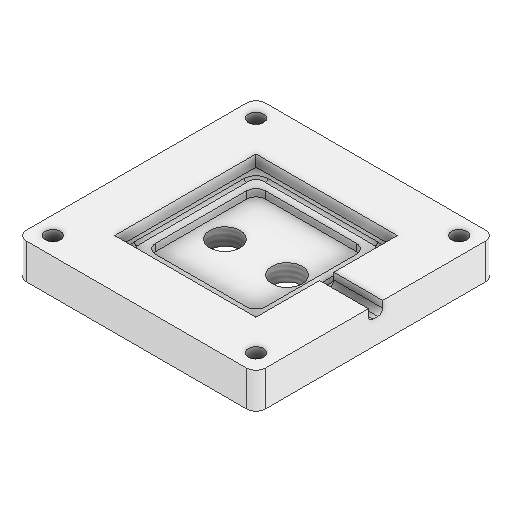
# Autodesk Inventor part: inf_soporte
Saved by Autodesk Inventor 2026.2 (Build 302298010, 298A)
## iProperties
Created: 2026-04-29
Part Number: inf_soporte
Material: Generic
Document SubType Name: Modeling
Designer: danie
Density: 1 g/cm^3
Appearance: Default
Author: danie
Autodesk Inventor part; units mm, degrees
ref_plane "YZ Plane" through (0, 0, 0) normal (1, 0, 0) x (0, 1, 0)
ref_plane "XZ Plane" through (0, 0, 0) normal (0, 1, 0) x (-1, 0, 0)
sketch "peltier" plane through (0, 0, 0) normal (0, 0, 1) x (1, 0, 0)
  line L0 (7.1779, -44.0485) -> (-50.9721, -44.0485)
  line L1 (-50.9721, -44.0485) -> (-50.9721, -102.2985)
  line L2 (-50.9721, -102.2985) -> (7.1779, -102.2985)
  line L3 (7.1779, -102.2985) -> (7.1779, -44.0485)
  point P0 (-21.8971, -73.1735)
  point P1 (-21.8971, -73.1735)
  dimension "d0" = 58.25
  dimension "d1" = 58.15
  measures "d0" distance between parallel lines of L2 L0
  measures "d1" distance between parallel lines of L3 L1
sketch "Sketch1" plane through (0, 0, 0) normal (0, 1, 0) x (-1, 0, 0)
  line L0 (-46, 50) -> (46, 50)
  line L1 (50, 46) -> (50, -46)
  line L2 (46, -50) -> (-46, -50)
  line L3 (-50, -46) -> (-50, 46)
  line L4 (-50, 50) -> (50, -50) construction
  line L5 (50, 50) -> (-50, -50) construction
  line L6 (-29.575, 29.575) -> (29.575, 29.575)
  line L7 (29.575, 29.575) -> (29.575, -29.575)
  line L8 (29.575, -29.575) -> (-29.575, -29.575)
  line L9 (-29.575, -29.575) -> (-29.575, 29.575)
  line L10 (-29.575, 29.575) -> (29.575, -29.575) construction
  line L11 (29.575, 29.575) -> (-29.575, -29.575) construction
  line L12 (-29.575, 0) -> (-50, 0)
  line L13 (-19, 23) -> (19, 23)
  line L14 (23, 19) -> (23, -19)
  line L15 (19, -23) -> (-19, -23)
  line L16 (-23, -19) -> (-23, 19)
  line L17 (-23, 23) -> (23, -23) construction
  line L18 (23, 23) -> (-23, -23) construction
  arc A0 (50, 46) -> (46, 50) centre (46, 46) ccw
  arc A1 (-46, 50) -> (-50, 46) centre (-46, 46) ccw
  arc A2 (-50, -46) -> (-46, -50) centre (-46, -46) ccw
  arc A3 (46, -50) -> (50, -46) centre (46, -46) ccw
  arc A4 (23, 19) -> (19, 23) centre (19, 19) ccw
  arc A5 (-19, 23) -> (-23, 19) centre (-19, 19) ccw
  arc A6 (-23, -19) -> (-19, -23) centre (-19, -19) ccw
  arc A7 (19, -23) -> (23, -19) centre (19, -19) ccw
  line L19 (-29.575, 0) -> (-29.575, -3)
  line L20 (-29.575, -3) -> (-50, -3)
  line L21 (-50, -3) -> (-50, 3)
  line L22 (-50, 3) -> (-29.575, 3)
  line L23 (-29.575, 3) -> (-29.575, -3)
  circle A8 centre (13, 0) radius 6.35
  circle A9 centre (-13, 0) radius 6.35
  line L24 (29.075, 29.125) -> (-29.075, 29.125)
  line L25 (-29.075, 29.125) -> (-29.075, -29.125)
  line L26 (-29.075, -29.125) -> (29.075, -29.125)
  line L27 (29.075, -29.125) -> (29.075, 29.125)
  point P0 (0, 0)
  point P1 (0, 0)
  dimension "d2" = 100
  dimension "d3" = 100
  dimension "d4" = 0.5
  dimension "d5" = 4
  dimension "d6" = 46
  dimension "d7" = 46
  dimension "d8" = 4
  dimension "d13" = 3
  dimension "d14" = 6
  dimension "d17" = 12.7
  dimension "d18" = 13
  dimension "d19" = 13
  dimension "d20" = 12.7
  constraints: 48 end point, 21 point on line, 16 point on circle, 16 tangent, 10 centre point, 8 midpoint, 6 equal radius, 6 parallel, 6 perpendicular, 3 horizontal, 2 other
  measures "d2" distance between parallel lines of L3 L1
  measures "d3" distance between parallel lines of L2 L0
  measures "d5" radius of A0
  measures "d6" distance between parallel lines of L16 L14
  measures "d7" distance between parallel lines of L13 L15
  measures "d8" radius of A4
  measures "d13" distance of L12.start L19.end
  measures "d14" distance of L20.end L21.end
  measures "d17" diameter of A8
  measures "d20" diameter of A9
extrude "Extrusion1" add sketch "Sketch1" along normal blind 20 contours L0 A0 L1 A3 L2 A2 L3 L20 L9 L8 L7 L6 L22 A1
extrude "Extrusion2" add sketch "Sketch1" along normal blind 15 contours L22 L9 L12 L3 | L12 L9 L20 L3 | L9 L6 L7 L8 | L27 L26 L25 L24
extrude "Extrusion3" add sketch "Sketch1" along normal blind 12 contours L13 A4 L14 A7 L15 A6 L16 A5
sketch "Sketch2" plane through (0, 15, 0) normal (0, 1, 0) x (1, 0, 0)
  line L0 (-29.575, -29.575) -> (-29.575, 29.575) projected
  line L1 (29.575, -29.575) -> (-29.575, -29.575) projected
  line L2 (29.575, -3) -> (29.575, -29.575) projected
  line L3 (50, -3) -> (29.575, -3) projected
  line L4 (50, -3) -> (50, 3) projected
  line L5 (29.575, 3) -> (50, 3) projected
  line L6 (29.575, 29.575) -> (29.575, 3) projected
  line L7 (-29.575, 29.575) -> (29.575, 29.575) projected
  line L8 (23, 19) -> (23, -19) projected
  arc A0 (19, -23) -> (23, -19) centre (19, -19) ccw projected
  line L9 (19, -23) -> (-19, -23) projected
  arc A1 (-23, -19) -> (-19, -23) centre (-19, -19) ccw projected
  line L10 (-23, -19) -> (-23, 19) projected
  arc A2 (-19, 23) -> (-23, 19) centre (-19, 19) ccw projected
  line L11 (-19, 23) -> (19, 23) projected
  arc A3 (23, 19) -> (19, 23) centre (19, 19) ccw projected
  line L12 (23, -27) -> (-23, -27)
  line L13 (-27, -23) -> (-27, 23)
  line L14 (-23, 27) -> (23, 27)
  line L15 (27, 23) -> (27, -23)
  line L16 (27, -27) -> (-27, 27) construction
  line L17 (-27, -27) -> (27, 27) construction
  arc A4 (-27, -23) -> (-23, -27) centre (-23, -23) ccw
  arc A5 (-23, 27) -> (-27, 23) centre (-23, 23) ccw
  arc A6 (27, 23) -> (23, 27) centre (23, 23) ccw
  arc A7 (23, -27) -> (27, -23) centre (23, -23) ccw
  point P0 (0, 0)
  dimension "d21" = 4
  dimension "d25" = 4
  dimension "d29" = 4
  constraints: 12 end point, 8 point on circle, 8 point on line, 8 tangent, 4 centre point, 3 equal radius, 2 midpoint, 2 parallel, 1 horizontal, 1 perpendicular
  measures "d21" distance between parallel lines of L10 L13
  measures "d25" radius of A4
  measures "d29" distance between parallel lines of L9 L12
ref_plane "Work Plane2" through (-27, 15, 23) normal (0, 0, -1) x (-1, 0, 0)
sketch "Sketch4" plane through (-27, 15, 23) normal (0, 0, -1) x (-1, 0, 0)
  circle A0 centre (0, 0) radius 1
  point P0 (-27, -15)
  dimension "d26" = 2
  constraints: 1 centre point
  measures "d26" diameter of A0
sweep "Sweep2" cut profiles "Sketch4" path "Sketch2" path curves L13 A5 L14 A6 L15 A7 L12 A4
thread "Thread1"
thread "Thread2"
move faces "Move1" translate (0, 5, 0) faces at (-3.5828, 0, -35.3125)
move faces "Move2" translate (0, -0.2, 0) faces at (-43.1917, 20, 9.8583)
fillet "Fillet1" radius 2 2 edges at (39.7875, 15, 3) (39.7875, 15, -3)
sketch "Sketch6" plane through (-46, 19.8, -50) normal (0, 1, 0) x (1, 0, 0)
  line L0 (96, -96) -> (96, -53) projected
  line L1 (96, -53) -> (75.575, -53) projected
  line L2 (75.575, -53) -> (75.575, -79.575) projected
  line L3 (75.575, -79.575) -> (16.425, -79.575) projected
  line L4 (16.425, -79.575) -> (16.425, -20.425) projected
  line L5 (16.425, -20.425) -> (75.575, -20.425) projected
  line L6 (75.575, -20.425) -> (75.575, -47) projected
  line L7 (75.575, -47) -> (96, -47) projected
  line L8 (96, -47) -> (96, -4) projected
  arc A0 (96, -4) -> (92, 0) centre (92, -4) ccw projected
  line L9 (92, 0) -> (0, 0) projected
  arc A1 (0, 0) -> (-4, -4) centre (0, -4) ccw projected
  line L10 (-4, -4) -> (-4, -96) projected
  arc A2 (-4, -96) -> (0, -100) centre (0, -96) ccw projected
  line L11 (0, -100) -> (92, -100) projected
  arc A3 (92, -100) -> (96, -96) centre (92, -96) ccw projected
  line L12 (3.5, -92.5) -> (88.5, -92.5)
  line L13 (88.5, -92.5) -> (88.5, -7.5)
  line L14 (88.5, -7.5) -> (3.5, -7.5)
  line L15 (3.5, -7.5) -> (3.5, -92.5)
  line L16 (3.5, -92.5) -> (88.5, -7.5) construction
  line L17 (88.5, -92.5) -> (3.5, -7.5) construction
  circle A4 centre (3.5, -92.5) radius 3.175
  circle A5 centre (3.5, -7.5) radius 3.175
  circle A6 centre (88.5, -92.5) radius 3.175
  circle A7 centre (88.5, -7.5) radius 3.175
  point P0 (46, -50)
  dimension "d43" = 6.35
  dimension "d45" = 85
  dimension "d46" = 85
  dimension "d49" = 85
  dimension "d52" = 85
  constraints: 12 end point, 4 centre point, 2 horizontal, 2 midpoint, 2 parallel, 1 coincident, 1 perpendicular, 1 vertical, 6 other
  measures "d43" diameter of A4
  measures "d45" distance between parallel lines of L14 L12
  measures "d46" distance between parallel lines of L13 L15
  measures "d49" distance of A4.centre A5.centre
  measures "d52" distance of A4.centre A6.centre
extrude "Extrusion4" cut sketch "Sketch6" against normal up to surface (14.8 mm away) contours A6 L12 L13 | L13 L12 A6 | A7 L14 L13 | L13 L14 A7 | A4 L15 L12 | L12 L15 A4 | A5 L15 L14 | L14 L15 A5
body "Solid1"
